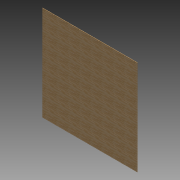
# Autodesk Inventor part: ground plne
Saved by Autodesk Inventor 2012 (Build 160160000, 160)
## iProperties
Created: 2012-03-08
Part Number: ground plne
Material: Default
Document SubType Name: Modeling
Designer: esv
Density: 1 g/cm^3
Author: esv
Autodesk Inventor part; units mm, degrees
ref_plane "YZ Plane" through (0, 0, 0) normal (1, 0, 0) x (0, 1, 0)
ref_plane "XZ Plane" through (0, 0, 0) normal (0, 1, 0) x (-1, 0, 0)
ref_plane "XY Plane" through (0, 0, 0) normal (0, 0, 1) x (1, 0, 0)
sketch "Sketch1" plane through (0, 0, 0) normal (0, 0, 1) x (1, 0, 0)
  line L0 (0, 0) -> (6096, 0)
  line L1 (6096, 0) -> (6096, 6096)
  line L2 (6096, 6096) -> (0, 6096)
  line L3 (0, 6096) -> (0, 0)
  dimension "d0" = 6096
  dimension "d1" = 6096
  constraints: 8 end point, 2 parallel, 1 horizontal, 1 perpendicular
  measures "d0" distance of L0.start L0.end
  measures "d1" distance of L2.end L0.start
extrude "Extrusion1" add sketch "Sketch1" along normal blind 25.4
body "Solid1"
